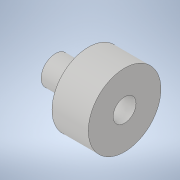
# Autodesk Inventor part: DTR-2
Saved by Autodesk Inventor 2021 (Build 250183000, 183)
## iProperties
Created: 2020-10-19
Part Number: DTR-2
Material: Generic
Document SubType Name: Modeling
Designer: Lucas Foulk
Density: 1 g/cm^3
Appearance: Default
Material_size: Tool Steel
Quantity: 3
Author: Lucas Foulk
Revision Number: 00
Autodesk Inventor part; units mm, degrees
ref_plane "YZ Plane" through (0, 0, 0) normal (1, 0, 0) x (0, 1, 0)
ref_plane "XZ Plane" through (0, 0, 0) normal (0, 1, 0) x (-1, 0, 0)
ref_plane "XY Plane" through (0, 0, 0) normal (0, 0, 1) x (1, 0, 0)
sketch "Sketch1" plane through (0, 0, 0) normal (1, 0, 0) x (0, 1, 0)
  circle A0 centre (0, 0) radius 5.0038
  circle A1 centre (0, 0) radius 4.0005
  dimension "d0" = 10.0076
  dimension "d1" = 8.001
  constraints: 2 centre point, 2 coincident
  measures "d0" diameter of A0
  measures "d1" diameter of A1
extrude "Extrusion1" add sketch "Sketch1" along normal blind 11.5062
sketch "Sketch2" plane through (11.5062, 0, 0) normal (1, 0, 0) x (0, 0, -1)
  circle A0 centre (0, 0) radius 12.7
  circle A1 centre (0, 0) radius 4.0005
  dimension "d4" = 25.4
  dimension "d7" = 8.001
  constraints: 2 centre point, 2 coincident
  measures "d4" diameter of A0
  measures "d7" diameter of A1
extrude "Extrusion2" add sketch "Sketch2" along normal blind 12.7
chamfer "Chamfer2" distance 0.254 angle 45 1 edges at (0, -4.0005, 0)
body "Solid1"
